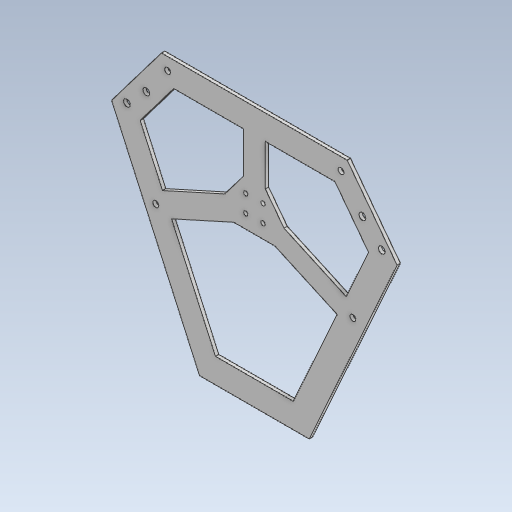
# Autodesk Inventor part: ChestMount
Saved by Autodesk Inventor 2020 (Build 240168000, 168)
## iProperties
Created: 2021-08-03
Part Number: ChestMount
Material: Generic
Document SubType Name: Sheet Metal
Designer: Val
Density: 1 g/cm^3
Sheet Metal Rule: Default
Appearance: Default
Author: Val
Autodesk Inventor part; units mm, degrees
ref_plane "YZ Plane" through (0, 0, 0) normal (1, 0, 0) x (0, 1, 0)
ref_plane "XZ Plane" through (0, 0, 0) normal (0, 1, 0) x (-1, 0, 0)
ref_plane "XY Plane" through (0, 0, 0) normal (0, 0, 1) x (1, 0, 0)
sketch "Base" plane through (0, 0, 0) normal (0, 0, 1) x (1, 0, 0)
  circle A0 centre (12.187819, 3.297819) radius 3.175
  circle A1 centre (-5.772693, -14.662693) radius 3.175
  circle A2 centre (212.394424, 3.297819) radius 3.175
  circle A3 centre (230.354936, -14.662693) radius 3.175
  arc A4 (-21.168075, -17.047312) -> (9.622688, 23.64295) centre (-130.364106, 97.577494) ccw construction
  arc A5 (214.959555, 23.64295) -> (245.750318, -17.047312) centre (354.946349, 97.577494) ccw construction
  line L0 (26.243247, 41.397819) -> (-19.976862, -19.682458)
  line L1 (12.187819, 3.297819) -> (212.394424, 3.297819) construction
  line L2 (112.291121, 41.397819) -> (112.291121, -199.902181) construction
  line L3 (26.243247, 41.397819) -> (112.291121, 41.397819)
  line L4 (-19.976862, -19.682458) -> (61.491121, -199.902181)
  line L5 (61.491121, -199.902181) -> (112.291121, -199.902181)
  line L6 (9.622688, 23.64295) -> (-21.168075, -17.047312) construction
  line L7 (-19.976862, -19.682458) -> (-21.168075, -17.047312) construction
  line L8 (62.346745, -145.552947) -> (162.235762, -145.552947) construction
  line L9 (89.431121, 18.537819) -> (89.431121, -177.042181) construction
  line L10 (89.431121, -177.042181) -> (76.244498, -177.042181)
  line L11 (76.244498, -177.042181) -> (6.449214, -22.644267)
  line L12 (6.449214, -22.644267) -> (37.612145, 18.537819)
  line L13 (37.612145, 18.537819) -> (89.431121, 18.537819)
  line L14 (89.431121, 18.537819) -> (112.291121, 18.537819)
  line L15 (89.431121, -177.042181) -> (112.291121, -177.042181)
  line L16 (198.338996, 41.397819) -> (244.559105, -19.682458)
  line L17 (198.338996, 41.397819) -> (112.291121, 41.397819)
  line L18 (244.559105, -19.682458) -> (163.091121, -199.902181)
  line L19 (163.091121, -199.902181) -> (112.291121, -199.902181)
  line L20 (135.151121, -177.042181) -> (148.337745, -177.042181)
  line L21 (148.337745, -177.042181) -> (218.133029, -22.644267)
  line L22 (218.133029, -22.644267) -> (186.970097, 18.537819)
  line L23 (186.970097, 18.537819) -> (135.151121, 18.537819)
  line L24 (135.151121, 18.537819) -> (112.291121, 18.537819)
  line L25 (135.151121, -177.042181) -> (112.291121, -177.042181)
  point P0 (0, 0)
  point P1 (112.291121, 3.297819)
extrude "Plate1" add sketch "Base" along normal blind 3.048
sketch "Sketch2" plane through (0, 0, 3.048) normal (0, 0, 1) x (1, 0, 0)
  circle A0 centre (104.291121, -48.262182) radius 2.05
  circle A1 centre (104.291121, -32.262181) radius 2.05
  circle A2 centre (120.291122, -32.262181) radius 2.05
  circle A3 centre (120.291122, -48.262182) radius 2.05
  line L0 (120.291122, -32.262181) -> (104.291121, -32.262181) construction
  line L1 (104.291121, -32.262181) -> (104.291121, -48.262182) construction
  line L2 (104.291121, -48.262182) -> (120.291122, -48.262182) construction
  line L3 (120.291122, -48.262182) -> (120.291122, -32.262181) construction
  line L4 (186.970097, 18.537819) -> (37.612145, 18.537819)
  line L5 (148.337745, -177.042181) -> (76.244498, -177.042181)
  line L6 (112.291121, 18.537819) -> (112.291121, -177.042181) construction
  line L7 (76.244498, -177.042181) -> (148.337745, -177.042181)
  line L8 (122.451121, 18.537819) -> (122.451121, -19.562181)
  line L9 (122.451121, -19.562181) -> (139.767673, -42.446156)
  line L10 (139.767673, -42.446156) -> (197.403821, -68.500466)
  line L11 (218.133029, -22.644267) -> (148.337745, -177.042181)
  line L12 (189.033686, -87.016493) -> (131.397539, -60.962182)
  line L13 (131.397539, -60.962182) -> (112.291121, -60.962182)
  line L14 (218.133029, -22.644267) -> (186.970097, 18.537819)
  line L15 (148.337745, -177.042181) -> (218.133029, -22.644267)
  line L16 (122.451121, -19.562181) -> (112.291121, -19.562181) construction
  line L17 (139.767673, -42.446156) -> (131.397539, -60.962182) construction
  line L18 (102.131121, 18.537819) -> (102.131121, -19.562181)
  line L19 (102.131121, -19.562181) -> (84.81457, -42.446156)
  line L20 (84.81457, -42.446156) -> (27.178422, -68.500466)
  line L21 (35.548557, -87.016493) -> (93.184704, -60.962182)
  line L22 (93.184704, -60.962182) -> (112.291121, -60.962182)
  line L23 (122.451121, 18.537819) -> (102.131121, 18.537819)
  line L24 (197.403821, -68.500466) -> (189.033686, -87.016493)
  line L25 (27.178422, -68.500466) -> (35.548557, -87.016493)
  line L26 (76.244498, -177.042181) -> (6.449214, -22.644267)
  point P0 (0, 0)
  point P1 (112.291121, -32.262181)
  dimension "d8" = 16
  dimension "d9" = 16
  dimension "d10" = 50.8
  dimension "d11" = 10.16
  dimension "d12" = 20.32
  dimension "d13" = 12.7
  dimension "d14" = 12.7
  measures "d8" distance of L0.start L0.end
  measures "d9" distance of L0.end L1.end
  measures "d10" distance between parallel lines of L0 L4
  measures "d11" distance between parallel lines of L6 L8
  measures "d12" distance between parallel lines of L12 L10
  measures "d13" distance between parallel lines of L16 L0
  measures "d14" distance between parallel lines of L2 L13
sheet face with bend "Face2" sketch "Sketch2" thickness 3.048 toward (0, 0, -1) bend radius 3.048 contours L8 L9 L10 L11 L12 L13 L22 L21 L25 L20 L19 L18 L4
bend "Bend1"
sketch "Sketch3" plane through (0, 0, 3.048) normal (0, 0, 1) x (1, 0, 0)
  circle A0 centre (31.927696, 29.967819) radius 2.794
  line L0 (26.243247, 41.397819) -> (-19.976862, -19.682458)
  line L1 (6.449214, -22.644267) -> (37.612145, 18.537819)
  line L2 (26.243247, 41.397819) -> (37.612145, 18.537819) construction
  line L3 (186.970097, 18.537819) -> (218.133029, -22.644267)
  line L4 (244.559105, -19.682458) -> (198.338996, 41.397819)
  line L5 (186.970097, 18.537819) -> (198.338996, 41.397819) construction
  circle A1 centre (192.654547, 29.967819) radius 2.794
  line L6 (27.178422, -68.500466) -> (6.449214, -22.644267)
  line L7 (27.178422, -68.500466) -> (35.548557, -87.016493) construction
  line L8 (31.36349, -77.75848) -> (10.53296, -87.174881) construction
  line L9 (61.491121, -199.902181) -> (-19.976862, -19.682458)
  circle A2 centre (20.948225, -82.466681) radius 2.794
  line L10 (26.243247, 41.397819) -> (198.338996, 41.397819)
  line L11 (112.291121, 41.397819) -> (112.291121, -60.962182) construction
  line L12 (93.184704, -60.962182) -> (131.397539, -60.962182)
  circle A3 centre (203.634018, -82.466681) radius 2.794
  point P0 (0, 0)
  dimension "d20" = 5.588
  dimension "d21" = 5.588
  constraints: 10 end point, 6 midpoint, 4 centre point, 2 coincident, 1 equal radius, 1 perpendicular, 1 point on line, 1 symmetric about line, 1 other
  measures "d20" diameter of A0
  measures "d21" diameter of A2
hole "Hole1" at (31.927696, 29.967819, 3.048) at (192.654547, 29.967819, 3.048) at (20.948225, -82.466681, 3.048) at (203.634018, -82.466681, 3.048) direction (0, 0, -1) diameter 5.588 end through all
equation "\"d12\" = 2 * d11"
equation "\"d27\" = Thickness"
equation "\"d7\" = Thickness"
equation "\"d15\" = BendRadius"
equation "\"d16\" = BendReliefWidth"
equation "\"d18\" = MinimumRemnant"
equation "\"d17\" = BendReliefDepth"
equation "\"d19\" = TransitionRadius"
equation "\"BendRadius\" = Thickness"
equation "\"BendReliefWidth\" = Thickness"
equation "\"BendReliefDepth\" = 0.5 * Thickness"
equation "\"CornerReliefSize\" = 4 * Thickness"
equation "\"MinimumRemnant\" = 2 * Thickness"
equation "\"TransitionRadius\" = BendRadius"
equation "\"JacobiRadiusSize\" = BendRadius"
equation "\"GapSize\" = Thickness"
equation "\"Thickness\" = 3.048"
body "Solid1"
